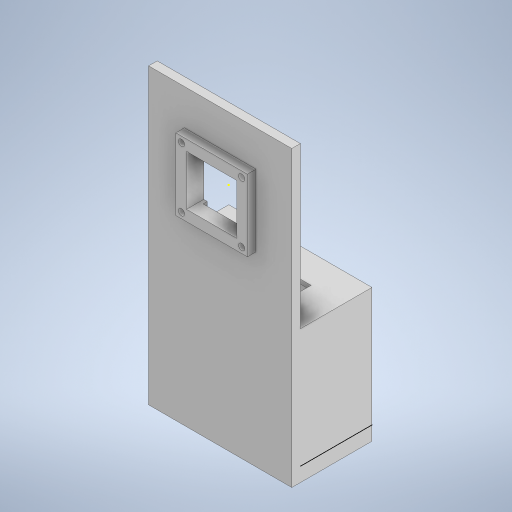
# Autodesk Inventor part: 12
Saved by Autodesk Inventor 2024 (Build 280153000, 153)
## iProperties
Created: 2025-12-09
Part Number: 12
Material: 常规
Document SubType Name: Modeling
Designer: 29555
Density: 1 g/cm^3
Appearance: 默认
Author: 29555
Autodesk Inventor part; units mm, degrees
ref_plane "YZ Plane" through (0, 0, 0) normal (1, 0, 0) x (0, 1, 0)
ref_plane "XZ Plane" through (0, 0, 0) normal (0, 1, 0) x (-1, 0, 0)
ref_plane "XY Plane" through (0, 0, 0) normal (0, 0, 1) x (1, 0, 0)
sketch "草图1" plane through (0, 0, 0) normal (0, 0, 1) x (1, 0, 0)
  line L0 (-50, -50) -> (50, -50)
  line L1 (50, -50) -> (50, 50)
  line L2 (50, 50) -> (-50, 50)
  line L3 (-50, 50) -> (-50, -50)
  line L4 (-50, -50) -> (50, 50) construction
  line L5 (50, -50) -> (-50, 50) construction
  line L6 (-50, -50) -> (50, -50)
  line L7 (50, -50) -> (50, -65)
  line L8 (50, -65) -> (-50, -65)
  line L9 (-50, -65) -> (-50, -50)
  point P0 (0, 0)
  dimension "d0" = 100
  dimension "d1" = 100
  dimension "d2" = 15
  constraints: 20 end point, 4 parallel, 2 horizontal, 2 midpoint, 2 perpendicular
  measures "d0" distance of L1.end L2.end
  measures "d1" distance of L0.end L1.end
  measures "d2" distance of L6.end L7.end
extrude "拉伸1" add sketch "草图1" along normal blind 6
sketch "草图2" plane through (0, 0, 6) normal (0, 0, 1) x (1, 0, 0)
  line L0 (-25, -25) -> (25, -25)
  line L1 (25, -25) -> (25, 25)
  line L2 (25, 25) -> (-25, 25)
  line L3 (-25, 25) -> (-25, -25)
  line L4 (-25, -25) -> (25, 25) construction
  line L5 (25, -25) -> (-25, 25) construction
  point P0 (0, 0)
  dimension "d5" = 50
  dimension "d6" = 50
  constraints: 12 end point, 2 midpoint, 2 parallel, 1 horizontal, 1 perpendicular
  measures "d5" distance of L1.end L2.end
  measures "d6" distance of L0.end L1.end
extrude "拉伸2" add sketch "草图2" along normal blind 6
sketch "草图3" plane through (0, 0, 12) normal (0, 0, 1) x (1, 0, 0)
  line L0 (-17.5, -17.5) -> (17.5, -17.5)
  line L1 (17.5, -17.5) -> (17.5, 17.5)
  line L2 (17.5, 17.5) -> (-17.5, 17.5)
  line L3 (-17.5, 17.5) -> (-17.5, -17.5)
  line L4 (-17.5, -17.5) -> (17.5, 17.5) construction
  line L5 (17.5, -17.5) -> (-17.5, 17.5) construction
  point P0 (0, 0)
  dimension "d9" = 35
  dimension "d10" = 35
  constraints: 12 end point, 2 midpoint, 2 parallel, 1 horizontal, 1 perpendicular
  measures "d9" distance of L1.end L2.end
  measures "d10" distance of L0.end L1.end
extrude "拉伸3" cut sketch "草图3" against normal through all
sketch "草图4" plane through (0, 0, 12) normal (0, 0, 1) x (1, 0, 0)
  line L0 (-21, -21) -> (21, -21)
  line L1 (21, -21) -> (21, 21)
  line L2 (21, 21) -> (-21, 21)
  line L3 (-21, 21) -> (-21, -21)
  line L4 (-21, -21) -> (21, 21) construction
  line L5 (21, -21) -> (-21, 21) construction
  circle A0 centre (21, 21) radius 2.15
  circle A1 centre (-21, 21) radius 2.15
  circle A2 centre (-21, -21) radius 2.15
  circle A3 centre (21, -21) radius 2.15
  point P0 (0, 0)
  dimension "d13" = 42
  dimension "d14" = 42
  dimension "d15" = 4.3
  dimension "d16" = 4.3
  dimension "d17" = 4.3
  dimension "d18" = 4.3
  constraints: 12 end point, 4 centre point, 4 coincident, 2 midpoint, 2 parallel, 1 horizontal, 1 perpendicular
  measures "d13" distance of L1.end L2.end
  measures "d14" distance of L0.end L1.end
  measures "d15" diameter of A1
  measures "d16" diameter of A0
  measures "d17" diameter of A3
  measures "d18" diameter of A2
extrude "拉伸4" cut sketch "草图4" against normal through all contours L3 A2 L0 | L0 A2 L3 | A3 L1 L0 | L0 L1 A3 | A1 L2 L3 | L3 L2 A1 | A0 L2 L1 | L1 L2 A0
sketch "草图5" plane through (0, 0, 0) normal (0, 0, -1) x (-1, 0, 0)
  line L0 (0, 0) -> (15, 0)
  line L1 (15, -17.5) -> (15, -57.5)
  line L2 (15, -57.5) -> (0, -57.5)
  line L3 (-17.5, -17.5) -> (17.5, -17.5) projected
  line L4 (15, -17.5) -> (0, -17.5)
  line L5 (-15, -17.5) -> (-15, -57.5)
  line L6 (-15, -57.5) -> (0, -57.5)
  line L7 (17.5, -17.5) -> (-17.5, -17.5)
  line L8 (0, -57.5) -> (10, -57.5)
  line L9 (10, -57.5) -> (10, -76.7389)
  line L10 (10, -76.7389) -> (0, -76.7389)
  line L11 (0, -76.7389) -> (0, -57.5)
  line L12 (-10, -57.5) -> (-10, -76.7389)
  line L13 (-10, -76.7389) -> (0, -76.7389)
  dimension "d21" = 15
  dimension "d22" = 40
  dimension "d23" = 10
  constraints: 26 end point, 3 parallel, 2 horizontal, 2 perpendicular, 2 point on line, 2 symmetric about line, 1 midpoint
  measures "d21" distance of L0.start L0.end
  measures "d22" distance of L1.start L1.end
  measures "d23" distance of L9.end L10.end
extrude "拉伸5" cut sketch "草图5" against normal blind 3
sketch "草图6" plane through (0, 0, 0) normal (0, 0, -1) x (-1, 0, 0)
  point P0 (0, 0)
sketch "草图7" plane through (-50, -65, 6) normal (0, -1, 0) x (1, 0, 0)
  line L0 (100, -6) -> (0, -6) projected
  line L1 (0, -6) -> (0, 0) projected
  line L2 (100, -6) -> (0, -6)
  line L3 (0, -6) -> (0, 0)
  line L4 (0, 0) -> (100, 0)
  line L5 (100, 0) -> (100, -6)
  point P0 (50, -6)
  constraints: 8 end point, 2 parallel, 1 horizontal, 1 perpendicular
extrude "拉伸6" add sketch "草图7" along normal blind 80
sketch "草图8" plane through (0, 0, 0) normal (0, 0, -1) x (-1, 0, 0)
  line L0 (10, -65) -> (-10, -65) projected
  line L1 (50, 50) -> (50, -145) projected
  line L2 (0, -65) -> (50, -65)
  line L3 (50, -65) -> (50, -145)
  line L4 (50, -145) -> (0, -145)
  line L5 (0, -145) -> (0, -65)
  line L6 (-50, 50) -> (-50, -145)
  line L7 (0, -65) -> (-50, -65)
  line L8 (-50, -145) -> (0, -145)
  point P0 (0, 0)
  constraints: 14 end point, 3 symmetric about line, 2 parallel, 1 horizontal, 1 midpoint, 1 perpendicular
extrude "拉伸7" cut sketch "草图8" against normal blind 3
sketch "草图9" plane through (0, 0, 3) normal (0, 0, -1) x (-1, 0, 0)
  line L0 (-50, -145) -> (-50, -65) projected
  line L1 (-50, -65) -> (-47, -65)
  line L2 (-47, -65) -> (-47, -142)
  line L3 (-47, -155.7604) -> (-50, -155.7604)
  line L4 (-50, -145) -> (-50, -65)
  line L5 (50, 50) -> (50, -145) projected
  line L6 (50, -65) -> (47, -65)
  line L7 (47, -65) -> (47, -142)
  line L8 (47, -155.7604) -> (50, -155.7604)
  line L9 (50, -145) -> (50, -65)
  line L10 (-47, -142) -> (47, -142)
  line L11 (63.4475, -142) -> (63.4475, -145)
  line L12 (50, -145) -> (-50, -145)
  line L13 (-50, -145) -> (-50, -142)
  point P0 (0, 0)
  point P1 (50, -145)
  dimension "d30" = 3
  dimension "d31" = 3
  dimension "d32" = 3
  constraints: 24 end point, 6 parallel, 4 point on line, 3 horizontal, 3 perpendicular
  measures "d30" distance of L8.start L8.end
  measures "d31" distance of L3.end L3.start
  measures "d32" distance of L11.end L11.start
extrude "拉伸8" add sketch "草图9" along normal blind 50
sketch "草图10" plane through (0, 0, -47) normal (0, 0, -1) x (-1, 0, 0)
  line L0 (50, -65) -> (47, -65) projected
  line L1 (50, -145) -> (50, -65) projected
  line L2 (-50, 50) -> (-50, -145) projected
  line L3 (-50, -145) -> (50, -145)
  line L4 (50, -145) -> (50, -65)
  line L5 (50, -65) -> (-50, -65)
  line L6 (-50, -65) -> (-50, -145)
  point P0 (0, 0)
  constraints: 8 end point, 2 parallel, 1 horizontal, 1 perpendicular
extrude "拉伸9" add sketch "草图10" along normal blind 3
sketch "草图11" plane through (-50, 50, 0) normal (-1, 0, 0) x (0, 0, 1)
  line L0 (-42.728, -178.1257) -> (-27.728, -178.1257)
  line L1 (-27.728, -178.1257) -> (-27.728, -188.1257)
  line L2 (-27.728, -188.1257) -> (-42.728, -188.1257)
  line L3 (-42.728, -188.1257) -> (-42.728, -178.1257)
  point P0 (0, -50)
  dimension "d37" = 10
  dimension "d38" = 15
  constraints: 8 end point, 2 parallel, 1 horizontal, 1 perpendicular
  measures "d37" distance of L0.end L1.end
  measures "d38" distance of L0.start L0.end
extrude "拉伸10" cut sketch "草图11" against normal blind 3
sketch "草图12" plane through (-50, -145, 6) normal (0, -1, 0) x (1, 0, 0)
  line L0 (0, -56) -> (100, -56) projected
  line L1 (100, -6) -> (100, -56) projected
  line L2 (100, -6) -> (97, -6) projected
  line L3 (100, -6) -> (100, -56) projected
  line L4 (0, -56) -> (100, -56) projected
  line L5 (0, -6) -> (0, -56) projected
  line L6 (3, -6) -> (0, -6) projected
  line L7 (3, -6) -> (3, -53) projected
  line L8 (3, -53) -> (97, -53) projected
  line L9 (97, -6) -> (97, -53) projected
  line L10 (100, -56) -> (0, -56)
  line L11 (0, -56) -> (0, -6)
  line L12 (0, -6) -> (100, -6)
  line L13 (100, -6) -> (100, -56)
  point P0 (50, -6)
  constraints: 8 end point, 2 parallel, 1 horizontal, 1 perpendicular
sketch "草图13" plane through (0, 0, -50) normal (0, 0, -1) x (-1, 0, 0)
  line L0 (50, -145) -> (50, -65) projected
  line L1 (50, -65) -> (-50, -65)
  line L2 (-53.2797, -65) -> (-53.2797, -62)
  line L3 (-50, -62) -> (50, -62)
  line L4 (50, -62) -> (50, -65)
  line L5 (-50, 50) -> (-50, -65) projected
  line L6 (-50, -62) -> (-50, -65)
  line L7 (-50, 50) -> (-50, -65) projected
  line L8 (-50, 50) -> (-50, -145) projected
  line L9 (-50, -65) -> (-50, -145) projected
  line L10 (-50, 50) -> (-50, -65) projected
  line L11 (-50, 50) -> (-50, -145) projected
  line L12 (-50, -65) -> (-50, -145) projected
  point P0 (0, 0)
  dimension "d41" = 3
  constraints: 10 end point, 2 parallel, 2 perpendicular, 1 horizontal, 1 point on line
  measures "d41" distance of L2.end L2.start
sketch "草图14" plane through (0, 0, 0) normal (0, 0, -1) x (-1, 0, 0)
  point P0 (0, 0)
extrude "拉伸11" add sketch "草图13" against normal blind 50
sketch "草图15" plane through (-50, -62, -50) normal (0, 1, 0) x (1, 0, 0)
  line L0 (50, -50) -> (35, -50)
  line L1 (35, -50) -> (35, -38)
  line L2 (35, -38) -> (50, -38)
  line L3 (50, -38) -> (50, -50)
  line L4 (50, -50) -> (65, -50)
  line L5 (65, -50) -> (65, -38)
  line L6 (65, -38) -> (50, -38)
  dimension "d44" = 15
  dimension "d45" = 12
  constraints: 14 end point, 2 parallel, 2 symmetric about line, 1 horizontal, 1 perpendicular
  measures "d44" distance of L1.end L2.end
  measures "d45" distance of L0.end L1.end
extrude "拉伸12" cut sketch "草图15" against normal blind 10
sketch "草图16" plane through (-50, -145, 6) normal (0, -1, 0) x (1, 0, 0)
  line L0 (50, -6) -> (50, -31)
  line L1 (100, -56) -> (0, -56) projected
  circle A0 centre (50, -31) radius 3.15
  dimension "d48" = 25
  dimension "d49" = 6.3
  constraints: 2 end point, 1 centre point, 1 coincident, 1 perpendicular
  measures "d48" distance of L0.start L0.end
  measures "d49" diameter of A0
extrude "拉伸13" cut sketch "草图16" against normal blind 10
sketch "草图17" plane through (0, 0, 12) normal (0, 0, 1) x (1, 0, 0)
  line L0 (17.5, 17.5) -> (-17.5, 17.5) projected
  line L1 (-17.5, -17.5) -> (17.5, -17.5)
  line L2 (17.5, -17.5) -> (17.5, 17.5)
  line L3 (17.5, 17.5) -> (-17.5, 17.5)
  line L4 (-17.5, 17.5) -> (-17.5, -17.5)
  line L5 (-17.5, -17.5) -> (17.5, 17.5) construction
  line L6 (17.5, -17.5) -> (-17.5, 17.5) construction
  line L7 (-12.5, -12.5) -> (12.5, -12.5)
  line L8 (12.5, -12.5) -> (12.5, 12.5)
  line L9 (12.5, 12.5) -> (-12.5, 12.5)
  line L10 (-12.5, 12.5) -> (-12.5, -12.5)
  line L11 (-12.5, -12.5) -> (12.5, 12.5) construction
  line L12 (12.5, -12.5) -> (-12.5, 12.5) construction
  point P0 (0, 0)
  dimension "d52" = 25
  dimension "d53" = 25
  constraints: 24 end point, 4 midpoint, 4 parallel, 2 horizontal, 2 perpendicular
  measures "d52" distance of L8.end L9.end
  measures "d53" distance of L7.end L8.end
extrude "拉伸14" add sketch "草图17" against normal blind 12
sketch "草图18" plane through (0, 0, 0) normal (0, 0, -1) x (-1, 0, 0)
  line L0 (-15, -17.5) -> (15, -17.5) projected
  line L1 (-15, -17.5) -> (15, -17.5)
  line L2 (15, -17.5) -> (15, -12.5)
  line L3 (15, -12.5) -> (-15, -12.5)
  line L4 (-15, -12.5) -> (-15, -17.5)
  point P0 (0, 0)
  point P1 (15, -17.5)
  dimension "d56" = 5
  constraints: 8 end point, 2 parallel, 1 horizontal, 1 perpendicular
  measures "d56" distance of L1.end L2.end
extrude "拉伸15" cut sketch "草图18" against normal blind 3
sketch "草图19" plane through (-50, -62, -50) normal (0, 1, 0) x (1, 0, 0)
  line L0 (35, -50) -> (35, -38) projected
  line L1 (35, -38) -> (65, -38) projected
  line L2 (65, -38) -> (65, -50) projected
  line L3 (100, -50) -> (65, -50) projected
  line L4 (100, 0) -> (100, -50) projected
  line L5 (0, 0) -> (100, 0) projected
  line L6 (0, 0) -> (0, -50) projected
  line L7 (35, -50) -> (0, -50) projected
  line L8 (35, -50) -> (35, -38) projected
  line L9 (35, -38) -> (65, -38) projected
  line L10 (65, -38) -> (65, -50) projected
  line L11 (100, -50) -> (65, -50) projected
  line L12 (100, 0) -> (100, -50) projected
  line L13 (0, 0) -> (100, 0) projected
  line L14 (0, 0) -> (0, -50) projected
  line L15 (35, -50) -> (0, -50) projected
  line L16 (50, -50) -> (77.5, -50)
  line L17 (77.5, -50) -> (77.5, -20)
  line L18 (77.5, -20) -> (50, -20)
  line L19 (50, -20) -> (50, -50)
  line L20 (50, -50) -> (22.5, -50)
  line L21 (22.5, -50) -> (22.5, -20)
  line L22 (22.5, -20) -> (50, -20)
  dimension "d59" = 27.5
  dimension "d60" = 30
  constraints: 14 end point, 2 parallel, 2 symmetric about line, 1 horizontal, 1 perpendicular
  measures "d59" distance of L17.end L18.end
  measures "d60" distance of L16.end L17.end
extrude "拉伸16" cut sketch "草图19" against normal blind 3 contours L7 L21 L22 L19 L1 L0 | L19 L18 L17 L3 L2 L1
sketch "草图20" plane through (-50, -145, 6) normal (0, -1, 0) x (1, 0, 0)
  circle A0 centre (50, -31) radius 3.15 projected
  circle A1 centre (50, -31) radius 3.15 projected
  line L0 (100, -56) -> (100, 0) projected
  line L1 (100, 0) -> (0, 0) projected
  line L2 (0, 0) -> (0, -56) projected
  line L3 (100, -56) -> (0, -56) projected
  circle A2 centre (50, -31) radius 3.15
  line L4 (100, -56) -> (0, -56)
  line L5 (0, -56) -> (0, 0)
  line L6 (0, 0) -> (100, 0)
  line L7 (100, 0) -> (100, -56)
  point P0 (50, -6)
  constraints: 8 end point, 2 parallel, 1 centre point, 1 coincident, 1 concentric, 1 horizontal, 1 perpendicular
extrude "拉伸17" add sketch "草图20" along normal blind 10
sketch "草图21" plane through (0, 0, 12) normal (0, 0, 1) x (1, 0, 0)
  line L0 (-17.5, -17.5) -> (17.5, -17.5)
  line L1 (17.5, -17.5) -> (17.5, 17.5)
  line L2 (17.5, 17.5) -> (-17.5, 17.5)
  line L3 (-17.5, 17.5) -> (-17.5, -17.5)
  line L4 (-17.5, -17.5) -> (17.5, 17.5) construction
  line L5 (17.5, -17.5) -> (-17.5, 17.5) construction
  point P0 (0, 0)
  dimension "d65" = 35
  dimension "d66" = 35
  constraints: 12 end point, 2 midpoint, 2 parallel, 1 horizontal, 1 perpendicular
  measures "d65" distance of L1.end L2.end
  measures "d66" distance of L0.end L1.end
extrude "拉伸18" cut sketch "草图21" against normal blind 15
sketch "草图22" plane through (0, 0, 0) normal (0, 0, -1) x (-1, 0, 0)
  point P0 (0, 0)
